6Fach_5mm_v3 (Autodesk Fusion 360 design; units mm, degrees)
Autodesk Fusion 360 part; units mm, degrees
cylinder "Grundkörper Zylinder1" add diameter 10 height 60 placed x (0, 0, -1) y (0, 1, 0) z (1, 0, 0) at (0, 0, 0) makes body 1
box "Grundkörper Quader1" add length 10 width 40 height 10 placed x (0, 0, 1) y (1, 0, 0) z (0, 1, 0) at (10, 0, -5) separate body makes body 2
cylinder "Grundkörper Zylinder3" cut diameter 4.5 height -10 placed x (1, 0, 0) y (0, 0, -1) z (0, 1, 0) at (15, 10, 0) bodies 1 2
cylinder "Grundkörper Zylinder4" cut diameter 4.5 height -10 placed x (1, 0, 0) y (0, 0, -1) z (0, 1, 0) at (25, 10, 0) bodies 1 2
cylinder "Grundkörper Zylinder5" cut diameter 4.5 height -10 placed x (1, 0, 0) y (0, 0, -1) z (0, 1, 0) at (35, 10, 0) bodies 1 2
cylinder "Grundkörper Zylinder6" cut diameter 4.5 height -10 placed x (1, 0, 0) y (0, 0, -1) z (0, 1, 0) at (45, 10, 0) bodies 1 2
cylinder "Grundkörper Zylinder7" cut diameter 5.3 height -7 placed x (1, 0, 0) y (0, 0, -1) z (0, 1, 0) at (15, 10, 0) bodies 1 2
cylinder "Grundkörper Zylinder8" cut diameter 5.3 height -7 placed x (1, 0, 0) y (0, 0, -1) z (0, 1, 0) at (25, 10, 0) bodies 1 2
cylinder "Grundkörper Zylinder9" cut diameter 5.3 height -7 placed x (1, 0, 0) y (0, 0, -1) z (0, 1, 0) at (35, 10, 0) bodies 1 2
cylinder "Grundkörper Zylinder10" cut diameter 5.3 height -7 placed x (1, 0, 0) y (0, 0, -1) z (0, 1, 0) at (45, 10, 0) bodies 1 2
cylinder "Grundkörper Zylinder11" cut diameter 4.5 height -65 placed x (0, 0, -1) y (0, 1, 0) z (1, 0, 0) at (60, 0, 0) bodies 1 2
extrude "Extrusion1" cut 1 faces at (60, -0.3602, -4.0563) along direction (-1, 0, 0) blind 5 on bodies 1 bodies 1
cylinder "Grundkörper Zylinder12" cut diameter 5.3 height -7 placed x (0, 0, -1) y (0, 1, 0) z (1, 0, 0) at (55, 0, 0) bodies 1 2
extrude "Extrusion2" cut 1 faces at (0, -0.3602, -4.0563) along direction (1, 0, 0) blind 5 on bodies 1 bodies 1
cylinder "Grundkörper Zylinder13" cut diameter 5.3 height -7 placed x (0, 0, 1) y (0, 1, 0) z (-1, 0, 0) at (5, 0, 0) bodies 1 2
fillet "Abrundung1" radius 0.7 16 edges at (5, -1.8081, 4.6616) (5, -2.4707, -0.9583) (55, 1.8081, 4.6616) (55, -2.4707, 0.9583) (50, 5, 5) (30, 10, 5) (50, 10, 0) (44.0417, 10, 2.4707) (34.0417, 10, 2.4707) (24.0417, 10, 2.4707) (14.0417, 10, 2.4707) (30, 10, -5) (10, 10, 0) (50, 5, -5) (10, 5, -5) (10, 5, 5) on bodies 1 2
sketch "Skizze16" plane through (0, 0, 0) normal (0, 1, 0) x (1, 0, 0)
  line L0 (10, 10) -> (16, 10)
  line L1 (16, 10) -> (16, 0)
  line L2 (16, 0) -> (10, 0)
  line L3 (10, 0) -> (10, 10)
  circle A0 centre (13, 10) radius 3
  circle A1 centre (13, 10) radius 1.75
  circle A2 centre (47, 10) radius 3
  line L4 (50, 10) -> (50, 0)
  line L5 (44, 0) -> (44, 10)
  line L6 (50, 0) -> (44, 0)
  circle A3 centre (47, 10) radius 1.75
  dimension "d37" = 3.5
  dimension "d38" = 3.5
  constraint horizontal L0
  constraint vertical L1
  constraint horizontal L2
  constraint vertical L3
  constraint midpoint L0 A0.centre
  constraint coincident L0.end A0
  constraint concentric A0 A1
  constraint vertical L4
  constraint horizontal L6
  constraint vertical L5
  constraint coincident L4.start A2
  constraint concentric A2 A3
  measures "d37" diameter of A1
  measures "d38" diameter of A3
extrude "Extrusion3" add sketch "Skizze16" against normal blind 2 separate body contours L0 A0 A1 | L0 A0 A1 | L1 L2 L3 A0 | A2 | A2 L4 L5 L6 makes body 3 at (47.0436, 0, -2.7516) makes body 4 at (13.0436, 0, -2.7516)
move_body "Verschieben1" bodies 4 3 to x (1, 0, 0) y (0, 1, 0) z (0, 0, 1) at (0, -3, 0)
fillet "Abrundung2" radius 0.3 8 faces at (45.7781, -4.3333, -8.7472) (49.7644, -4.3333, -11.1653) (50, -3.6667, -6.6667) (44, -3.6667, -3.3333) (14.7413, -4.3333, -10.1742) (10.0595, -4.3333, -10.5944) (16, -3.6667, -6.6667) (10, -3.6667, -3.3333) on bodies 3 4
